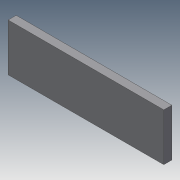
# Autodesk Inventor part: foot bracket foot backside
Saved by Autodesk Inventor 2019 (Build 230136000, 136)
## iProperties
Created: 2019-02-27
Part Number: foot bracket foot backside
Material: Generic
Document SubType Name: Modeling
Designer: LillaHunden
Density: 1 g/cm^3
Appearance: Default
Author: LillaHunden
Autodesk Inventor part; units mm, degrees
ref_plane "YZ Plane" through (0, 0, 0) normal (1, 0, 0) x (0, 1, 0)
ref_plane "XZ Plane" through (0, 0, 0) normal (0, 1, 0) x (-1, 0, 0)
ref_plane "XY Plane" through (0, 0, 0) normal (0, 0, 1) x (1, 0, 0)
sketch "Sketch1" plane through (0, 0, 0) normal (0, 0, 1) x (1, 0, 0)
  line L0 (148.5, -9.5) -> (148.5, -6.2) construction
  line L1 (148.5, -6.2) -> (193, -6.2) construction
  line L2 (193, 9.5) -> (193, -6.2) construction
  line L3 (0, 9.5) -> (193, 9.5) construction
  line L4 (0, -9.5) -> (0, 9.5) construction
  line L5 (148.5, -9.5) -> (0, -9.5) construction
  line L6 (0, 9.5) -> (193, 9.5)
  line L7 (193, 9.5) -> (193, -57.5)
  line L8 (193, -57.5) -> (0, -57.5)
  line L9 (0, -57.5) -> (0, 9.5)
  point P0 (0, 0)
  constraints: 8 end point, 2 parallel, 1 horizontal, 1 perpendicular
extrude "Extrusion1" add sketch "Sketch1" along normal blind 10
sketch "Sketch2" plane through (0, -57.5, 0) normal (-1, 0, 0) x (0, 0, 1)
  line L0 (-111.7541, 55) -> (-111.7541, 67) construction
  line L1 (-116, 67) -> (-111.7541, 67) construction
  line L2 (-116, 48) -> (-116, 67) construction
  line L3 (4, 48) -> (-116, 48) construction
  line L4 (4, 48) -> (4, 67) construction
  line L5 (-54.7541, 67) -> (4, 67) construction
  line L6 (-54.7541, 67) -> (-54.7541, 55) construction
  line L7 (-54.7541, 55) -> (-111.7541, 55) construction
  line L8 (0, 67) -> (0, 0) projected
  line L9 (4, 67) -> (0, 67)
  line L10 (0, 67) -> (0, 48)
  line L11 (0, 48) -> (4, 48)
  line L12 (4, 48) -> (4, 67)
  point P0 (0, 57.5)
  constraints: 8 end point, 2 parallel, 2 point on line, 1 horizontal, 1 perpendicular
extrude "Extrusion2" cut sketch "Sketch2" against normal through all
body "Solid1"
